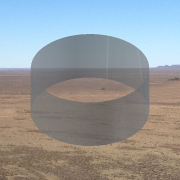
# Autodesk Inventor part: bpCylinder
Saved by Autodesk Inventor 2014 SP1 (Build 180222100, 222)
## iProperties
Created: 2015-05-04
Part Number: bpCylinder
Material: Glass
Document SubType Name: Modeling
Designer: Dave
Mass: 2301.13 g
Surface Area: 101216 cm^2
Volume: 1055.56 cm^3
Density: 2.18 g/cm^3
Appearance: Clear
Author: Dave
Autodesk Inventor part; units mm, degrees
ref_plane "YZ Plane" through (0, 0, 0) normal (1, 0, 0) x (0, 1, 0)
ref_plane "XZ Plane" through (0, 0, 0) normal (0, 1, 0) x (-1, 0, 0)
ref_plane "XY Plane" through (0, 0, 0) normal (0, 0, 1) x (1, 0, 0)
sketch "Sketch1" plane through (0, 0, 0) normal (0, 0, 1) x (1, 0, 0)
  line L0 (-1016, 0) -> (-1016.2086, 0)
  line L1 (-1016.2086, 0) -> (-1016.2086, 914.4)
  line L2 (-1016.2086, 914.4) -> (-1016, 914.4)
  line L3 (-1016, 914.4) -> (-1016, 0)
  line L4 (0, -182.88) -> (0, 1097.28) projected
  point P0 (0, 0)
  dimension "d0" = 914.4
  dimension "d1" = 1016
  constraints: 8 end point, 2 parallel, 1 horizontal, 1 perpendicular
  measures "d0" distance of L0.end L1.end
  measures "d1" distance of L0.start point (0, 0)
revolve "Revolution1" add sketch "Sketch1" angle 360 about axis through (0, -10, 0) along (0, 1, 0)
body "Solid1"
